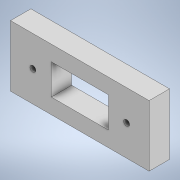
# Autodesk Inventor part: 1st arm closing
Saved by Autodesk Inventor 2022 (Build 260153000, 153)
## iProperties
Created: 2021-06-29
Part Number: 1st arm closing
Material: Generic
Document SubType Name: Modeling
Designer: USER
Density: 1 g/cm^3
Appearance: Default
Author: USER
Autodesk Inventor part; units mm, degrees
ref_plane "YZ Plane" through (0, 0, 0) normal (1, 0, 0) x (0, 1, 0)
ref_plane "XZ Plane" through (0, 0, 0) normal (0, 1, 0) x (-1, 0, 0)
ref_plane "XY Plane" through (0, 0, 0) normal (0, 0, 1) x (1, 0, 0)
sketch "Sketch1" plane through (0, 0, 0) normal (0, 0, 1) x (1, 0, 0)
  line L0 (-34, 15) -> (34, 15)
  line L1 (34, 15) -> (34, -15)
  line L2 (34, -15) -> (-34, -15)
  line L3 (-34, -15) -> (-34, 15)
  line L4 (-34, 15) -> (34, -15) construction
  line L5 (34, 15) -> (-34, -15) construction
  point P0 (0, 0)
  dimension "d0" = 68
  dimension "d1" = 30
  constraints: 12 end point, 2 midpoint, 2 parallel, 1 horizontal, 1 perpendicular
  measures "d0" distance of L1.end L2.end
  measures "d1" distance of L0.end L1.end
extrude "Extrusion1" add sketch "Sketch1" along normal blind 10
sketch "Sketch2" plane through (0, 0, 10) normal (0, 0, 1) x (1, 0, 0)
  line L0 (-14, 7.5) -> (14, 7.5)
  line L1 (14, 7.5) -> (14, -7.5)
  line L2 (14, -7.5) -> (-14, -7.5)
  line L3 (-14, -7.5) -> (-14, 7.5)
  line L4 (-14, 7.5) -> (14, -7.5) construction
  line L5 (14, 7.5) -> (-14, -7.5) construction
  point P0 (0, 0)
  dimension "d4" = 28
  dimension "d5" = 15
  constraints: 12 end point, 2 midpoint, 2 parallel, 1 horizontal, 1 perpendicular
  measures "d4" distance of L1.end L2.end
  measures "d5" distance of L0.end L1.end
extrude "Extrusion2" cut sketch "Sketch2" against normal blind 10
sketch "Sketch3" plane through (0, 0, 10) normal (0, 0, 1) x (1, 0, 0)
  circle A0 centre (-23, 0) radius 1.4515
  circle A1 centre (23, 0) radius 1.4515
  line L0 (-14, -7.5) -> (-14, 7.5) projected
  line L1 (14, 7.5) -> (14, -7.5) projected
  point P0 (0, 0)
  dimension "d8" = 2.903
  dimension "d9" = 2.903
  dimension "d10" = 9
  dimension "d11" = 9
  constraints: 2 centre point
  measures "d8" diameter of A0
  measures "d9" diameter of A1
  measures "d10" distance from line of L0 A0.centre
  measures "d11" distance from line of A1.centre L1
extrude "Extrusion3" cut sketch "Sketch3" against normal blind 10
body "Solid1"
